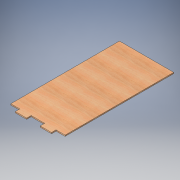
# Autodesk Inventor part: Bottom
Saved by Autodesk Inventor 2016 (Build 200138000, 138)
## iProperties
Created: 2016-02-10
Part Number: Bottom
Material: Wood (Birch)
Document SubType Name: Modeling
Designer: ron
Density: 0.55 g/cm^3
Appearance: Birch - Natural Polished
Author: ron
Autodesk Inventor part; units mm, degrees
ref_plane "YZ Plane" through (0, 0, 0) normal (1, 0, 0) x (0, 1, 0)
ref_plane "XZ Plane" through (0, 0, 0) normal (0, 1, 0) x (-1, 0, 0)
ref_plane "XY Plane" through (0, 0, 0) normal (0, 0, 1) x (1, 0, 0)
sketch "Sketch1" plane through (0, 0, 0) normal (0, 1, 0) x (-1, 0, 0)
  line L0 (609.6, 0) -> (609.6, -1219.2)
  line L1 (609.6, -1219.2) -> (0, -1219.2)
  line L2 (0, -1219.2) -> (0, 0)
  line L3 (609.6, 0) -> (508, 0)
  line L4 (508, 0) -> (508, 50.8)
  line L5 (508, 50.8) -> (381, 50.8)
  line L6 (381, 50.8) -> (381, 0)
  line L7 (381, 0) -> (228.6, 0)
  line L8 (228.6, 0) -> (228.6, 50.8)
  line L9 (228.6, 50.8) -> (101.6, 50.8)
  line L10 (101.6, 50.8) -> (101.6, 0)
  line L11 (508, 0) -> (609.6, 0)
  line L12 (0, 0) -> (101.6, 0)
  line L13 (228.6, 0) -> (381, 0)
  dimension "d0" = 1219.2
  dimension "d1" = 609.6
  dimension "d4" = 101.6
  dimension "d5" = 50.8
  dimension "d6" = 127
  dimension "d7" = 152.4
  dimension "d8" = 50.8
  dimension "d9" = 127
  constraints: 28 end point, 11 perpendicular, 4 parallel, 3 horizontal, 2 point on line
  measures "d0" distance of L0.start L0.end
  measures "d1" distance of L0.end L1.end
  measures "d4" distance of L0.start L3.end
  measures "d5" distance of L3.end L4.end
  measures "d6" distance of L4.end L5.end
  measures "d7" distance of L6.end L7.end
  measures "d8" distance of L7.end L8.end
  measures "d9" distance of L8.end L9.end
extrude "Extrusion1" add sketch "Sketch1" along normal blind 12.7
body "Solid1"
